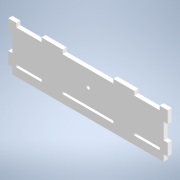
# Autodesk Inventor part: case bottom sides
Saved by Autodesk Inventor 2022 (Build 260153000, 153)
## iProperties
Created: 2021-05-28
Part Number: case bottom sides
Material: ABS Plastic
Document SubType Name: Modeling
Designer: benka
Density: 1.06 g/cm^3
Appearance: Smooth - White
Author: benka
Autodesk Inventor part; units mm, degrees
ref_plane "YZ Plane" through (0, 0, 0) normal (1, 0, 0) x (0, 1, 0)
ref_plane "XZ Plane" through (0, 0, 0) normal (0, 1, 0) x (-1, 0, 0)
ref_plane "XY Plane" through (0, 0, 0) normal (0, 0, 1) x (1, 0, 0)
sketch "Sketch1" plane through (0, 0, 0) normal (0, 0, 1) x (1, 0, 0)
  ellipse E0 centre (0, 0) end of major axis (1.9913, 0) minor radius 2.0309
  line L0 (93.7419, -25.0004) -> (98.7419, -25.0004)
  line L1 (98.7419, -25.0004) -> (98.7419, -10.0012)
  line L2 (93.7419, -10.0012) -> (98.7419, -10.0012)
  line L3 (93.7419, -10.0012) -> (93.7419, 9.9988)
  line L4 (93.7419, 9.9988) -> (98.7419, 9.9988)
  line L5 (98.7419, 9.9988) -> (98.7419, 25.0003)
  line L6 (-99.2581, 9.9988) -> (-99.2581, 25.0003)
  line L7 (-99.2581, 9.9988) -> (-94.2581, 9.9988)
  line L8 (-99.2581, -10.0012) -> (-99.2581, -25.0004)
  line L9 (-99.2581, -10.0012) -> (-94.2581, -10.0012)
  line L10 (-99.2581, -25.0004) -> (-94.2581, -25.0004)
  line L11 (-94.2581, 9.9988) -> (-94.2581, -10.0012)
  line L12 (-94.2581, -25.0004) -> (-94.2581, -33.0004)
  line L13 (93.7419, -33.0004) -> (93.7419, -25.0004)
  line L14 (-94.2581, -33.0004) -> (93.7419, -33.0004)
  line L15 (-89.2581, 25.0003) -> (-89.2581, 20.0003)
  line L16 (-89.2581, 20.0003) -> (-58.0081, 20.0003)
  line L17 (-58.0081, 25.0003) -> (-58.0081, 20.0003)
  line L18 (-58.0081, 25.0003) -> (-31.7581, 25.0003)
  line L19 (-31.7581, 25.0003) -> (-31.7581, 20.0003)
  line L20 (-31.7581, 20.0003) -> (31.2419, 20.0003)
  line L21 (31.2419, 25.0003) -> (31.2419, 20.0003)
  line L22 (31.2419, 25.0003) -> (57.4919, 25.0003)
  line L23 (57.4919, 25.0003) -> (57.4919, 20.0003)
  line L24 (57.4919, 20.0003) -> (88.7419, 20.0003)
  line L25 (88.7419, 25.0003) -> (88.7419, 20.0003)
  line L26 (-89.2581, 25.0003) -> (-99.2581, 25.0003)
  line L27 (88.7419, 25.0003) -> (98.7419, 25.0003)
  line L28 (88.7419, -20.0004) -> (57.4919, -20.0004)
  line L29 (57.4919, -20.0004) -> (57.4919, -23.0004)
  line L30 (57.4919, -23.0004) -> (88.7419, -23.0004)
  line L31 (88.7419, -23.0004) -> (88.7419, -20.0004)
  line L32 (31.2419, -20.0004) -> (-31.7581, -20.0004)
  line L33 (-31.7581, -20.0004) -> (-31.7581, -23.0004)
  line L34 (-31.7581, -23.0004) -> (31.2419, -23.0004)
  line L35 (31.2419, -23.0004) -> (31.2419, -20.0004)
  line L36 (-58.0081, -20.0004) -> (-89.2581, -20.0004)
  line L37 (-89.2581, -20.0004) -> (-89.2581, -23.0004)
  line L38 (-89.2581, -23.0004) -> (-58.0081, -23.0004)
  line L39 (-58.0081, -23.0004) -> (-58.0081, -20.0004)
  point P0 (-93.0453, -16.9364)
  dimension "d46" = 5
  constraints: 80 end point, 12 perpendicular, 8 horizontal, 6 parallel, 5 collinear, 5 vertical, 1 centre point, 1 point on line, 17 other
  measures "d46" distance between parallel lines of L24 L27
extrude "Extrusion3" add sketch "Sketch1" along normal blind 5
body "Solid3"
